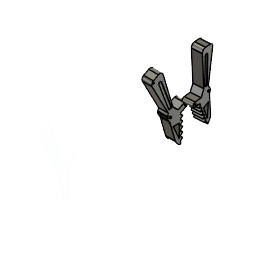
6DOF INDUSTRIAL ROBOTIC ARM (Autodesk Fusion 360 archive; units mm, degrees)
design "JAW 7:1"
part number: 2026-03-04-21-54-08-380
Autodesk Fusion 360 part; units mm, degrees
(part 1 of 2)
sketch "Sketch1" plane through (0, 0, 0) normal (1, 0, 0) x (0, 0, -1)
  line L0 (202.1362, -69.2043) -> (169.6449, -7.2018)
  line L1 (169.6449, -7.2018) -> (190.7116, 4.2958)
  line L2 (190.7116, 4.2958) -> (210.5911, -63.8644)
  line L3 (210.5911, -63.8644) -> (202.1362, -69.2043)
  line L4 (202.1362, -69.2043) -> (200.5414, -75)
  line L5 (200.5414, -75) -> (200.5414, -78.3577)
  line L6 (200.5414, -78.3577) -> (205, -85)
  line L7 (205, -85) -> (215, -120)
  line L8 (215, -120) -> (215, -130)
  line L9 (215, -130) -> (225, -130)
  line L10 (225, -130) -> (225, -80)
  line L11 (225, -80) -> (235, -75)
  line L12 (210.5911, -63.8644) -> (220, -72.7707)
  line L13 (220, -72.7707) -> (231.4715, -67.0349)
  arc A0 (235, -75) -> (231.1083, -67.2166) centre (233.2358, -71.0175) ccw
  dimension "d8" = 70
  dimension "d9" = 24
  dimension "d10" = 71
  dimension "d11" = 15
  dimension "d12" = 10
  dimension "d14" = 10
  dimension "d15" = 8
  dimension "d19" = 8.7116
  constraint vertical L5
  constraint vertical L8
  constraint perpendicular L8 L9
  constraint perpendicular L9 L10
  constraint parallel L11 L13
  constraint coincident L13.end A0
  constraint coincident L13 A0.end
  measures "d8" distance of L0.start L0.end
  measures "d9" distance of L0.end L1.end
  measures "d10" distance of L2.end L1.end
  measures "d11" distance of L2.end L4.end
  measures "d12" distance of L0.start L2.end
  measures "d14" vertical distance of L4.end L6.end
  measures "d15" distance of L5.end L6.end
  measures "d19" distance of L11.end L13.end
extrude "Extrude1" add sketch "Sketch1" along normal mid plane 18 contours L0 L1 L2 L3 | L3 L4 L5 L6 L7 L8 L9 L10 L11 L12 L13 A0 makes body 1
sketch "Sketch2" plane through (-9, 0, 0) normal (-1, 0, 0) x (0, 0, 1)
  line L0 (-200.5414, -75) -> (-202.1362, -69.2043)
  line L1 (-202.1362, -69.2043) -> (-169.6449, -7.2018)
  line L2 (-169.6449, -7.2018) -> (-190.7116, 4.2958)
  line L3 (-190.7116, 4.2958) -> (-210.5911, -63.8644)
  line L4 (-210.5911, -63.8644) -> (-220, -72.7707)
  line L5 (-220, -72.7707) -> (-231.4715, -67.0349)
  arc A0 (-231.4715, -67.0349) -> (-235, -75) centre (-233.2358, -71.0175) ccw
  line L6 (-235, -75) -> (-225, -80)
  line L7 (-225, -80) -> (-225, -130)
  line L8 (-225, -130) -> (-215, -130)
  line L9 (-215, -130) -> (-215, -120)
  line L10 (-215, -120) -> (-205, -85)
  line L11 (-205, -85) -> (-200.5414, -78.3577)
  line L12 (-200.5414, -78.3577) -> (-200.5414, -75)
sketch "Sketch3" plane through (9, 0, 0) normal (1, 0, 0) x (0, 0, -1)
  line L0 (202.1362, -69.2043) -> (200.5414, -75)
  line L1 (200.5414, -75) -> (200.5414, -78.3577)
  line L2 (200.5414, -78.3577) -> (205, -85)
  line L3 (205, -85) -> (215, -120)
  line L4 (215, -120) -> (215, -130)
  line L5 (215, -130) -> (225, -130)
  line L6 (225, -130) -> (225, -80)
  line L7 (225, -80) -> (235, -75)
  arc A0 (235, -75) -> (231.4715, -67.0349) centre (233.2358, -71.0175) ccw
  line L8 (231.4715, -67.0349) -> (220, -72.7707)
  line L9 (220, -72.7707) -> (210.5911, -63.8644)
  line L10 (210.5911, -63.8644) -> (190.7116, 4.2958)
  line L11 (190.7116, 4.2958) -> (169.6449, -7.2018)
  line L12 (169.6449, -7.2018) -> (202.1362, -69.2043)
  line L13 (215, -120) -> (222.3, -120)
  line L14 (222.3, -120) -> (222.3, -95)
  line L15 (222.3, -95) -> (211.3, -95)
  line L16 (211.3, -95) -> (222.3, -120)
  dimension "d23" = 25
  dimension "d24" = 11
  dimension "d25" = 2.7
  constraint coincident L3.end L4.start
  constraint perpendicular L4 L13
  constraint perpendicular L13 L14
  constraint perpendicular L14 L15
  measures "d23" distance of L13.end L14.end
  measures "d24" distance of L14.end L15.end
  measures "d25" distance of L6 L14
extrude "Extrude2" cut sketch "Sketch3" against normal blind 37 contours L14 L15 L16 bodies 1
sketch "Sketch4" plane through (9, 0, 0) normal (1, 0, 0) x (0, 0, -1)
  line L0 (222.3, -95) -> (222.3, -120)
  line L1 (222.3, -120) -> (211.3, -95)
  line L2 (211.3, -95) -> (222.3, -95)
  line L3 (202.1362, -69.2043) -> (200.5414, -75)
  line L4 (200.5414, -75) -> (200.5414, -78.3577)
  line L5 (200.5414, -78.3577) -> (205, -85)
  line L6 (205, -85) -> (215, -120)
  line L7 (215, -120) -> (215, -130)
  line L8 (215, -130) -> (225, -130)
  line L9 (225, -130) -> (225, -80)
  line L10 (225, -80) -> (235, -75)
  arc A0 (235, -75) -> (231.4715, -67.0349) centre (233.2358, -71.0175) ccw
  line L11 (231.4715, -67.0349) -> (220, -72.7707)
  line L12 (220, -72.7707) -> (210.5911, -63.8644)
  line L13 (210.5911, -63.8644) -> (190.7116, 4.2958)
  line L14 (190.7116, 4.2958) -> (169.6449, -7.2018)
  line L15 (169.6449, -7.2018) -> (202.1362, -69.2043)
  line L16 (225, -130) -> (225, -125)
  line L17 (225, -125) -> (225, -121)
  line L18 (225, -121) -> (229, -121)
  line L19 (225, -118) -> (229, -121)
  line L20 (229, -121) -> (225, -124)
  line L21 (225, -109.25) -> (229, -112.25)
  line L22 (229, -112.25) -> (225, -115.25)
  line L23 (225, -100.5) -> (229, -103.5)
  line L24 (229, -103.5) -> (225, -106.5)
  line L25 (225, -91.75) -> (229, -94.75)
  line L26 (229, -94.75) -> (225, -97.75)
  line L27 (225, -83) -> (229, -86)
  line L28 (229, -86) -> (225, -89)
  dimension "d28" = 5
  dimension "d29" = 4
  dimension "d30" = 4
  dimension "d35" = 0
  dimension "d36" = 35
  constraint coincident L8.end L9.start
  constraint perpendicular L8 L16
  constraint parallel L9 L17
  constraint perpendicular L9 L18
  constraint coincident L9 L19.start
  constraint coincident L9 L20.end
  measures "d28" distance of L8.end L16.end
  measures "d29" distance of L16.end L17.end
  measures "d30" distance of L17.end L18.end
extrude "Extrude3" add sketch "Sketch4" against normal up to surface (18 mm away) contours L9 L17 L18 L20 | L9 L18 L19 bodies 1
extrude "Extrude4" add sketch "Sketch4" against normal up to surface (18 mm away) contours L9 L27 L28 | L9 L25 L26 | L9 L21 L22 | L9 L23 L24 bodies 1
fillet "Fillet1" radius 6 2 edges at (0, 4.2958, -190.7116) (0, -7.2018, -169.6449) on bodies 1
fillet "Fillet2" radius 15 1 edges at (0, -130, -215) on bodies 1
fillet "Fillet3" radius 7.5 2 edges at (0, -75, -200.5414) (0, -78.3577, -200.5414) on bodies 1
sketch "Sketch5" plane through (9, 0, 0) normal (1, 0, 0) x (0, 0, -1)
  arc A0 (200.5414, -76.0739) -> (201.8142, -80.2539) centre (208.0414, -76.0739) ccw
  line L0 (201.8142, -80.2539) -> (205, -85)
  line L1 (205, -85) -> (215, -120)
  arc A1 (215, -120) -> (225, -130) centre (229.3541, -115.6459) ccw
  line L2 (225, -130) -> (225, -124)
  line L3 (225, -124) -> (229, -121)
  line L4 (229, -121) -> (225, -118)
  line L5 (225, -118) -> (225, -115.25)
  line L6 (225, -115.25) -> (229, -112.25)
  line L7 (229, -112.25) -> (225, -109.25)
  line L8 (225, -109.25) -> (225, -106.5)
  line L9 (225, -106.5) -> (229, -103.5)
  line L10 (229, -103.5) -> (225, -100.5)
  line L11 (225, -100.5) -> (225, -97.75)
  line L12 (225, -97.75) -> (229, -94.75)
  line L13 (229, -94.75) -> (225, -91.75)
  line L14 (225, -91.75) -> (225, -89)
  line L15 (225, -89) -> (229, -86)
  line L16 (229, -86) -> (225, -83)
  line L17 (225, -83) -> (225, -80)
  line L18 (225, -80) -> (235, -75)
  arc A2 (235, -75) -> (231.4715, -67.0349) centre (233.2358, -71.0175) ccw
  line L19 (231.4715, -67.0349) -> (220, -72.7707)
  line L20 (220, -72.7707) -> (210.5911, -63.8644)
  line L21 (210.5911, -63.8644) -> (192.7997, -2.8637)
  arc A3 (192.7997, -2.8637) -> (184.1653, 0.723) centre (187.0397, -4.5436) ccw
  line L22 (184.1653, 0.723) -> (174.8233, -4.3755)
  arc A4 (174.8233, -4.3755) -> (172.3832, -12.4272) centre (177.6977, -9.6422) ccw
  line L23 (172.3832, -12.4272) -> (202.1362, -69.2043)
  line L24 (202.1362, -69.2043) -> (200.8102, -74.0232)
  arc A5 (200.8102, -74.0232) -> (200.5414, -76.0131) centre (208.0414, -76.0131) ccw
  line L25 (200.5414, -76.0131) -> (200.5414, -76.0739)
  line L26 (222.3, -95) -> (222.3, -120)
  line L27 (222.3, -120) -> (211.3, -95)
  line L28 (211.3, -95) -> (222.3, -95)
  circle A6 centre (175, -8) radius 1.4142
extrude "Extrude5" cut sketch "Sketch5" against normal blind 15 contours A6 bodies 1
sketch "Sketch6" plane through (0, 47.7358, -167.0755) normal (0, -0.274721, 0.961524) x (1, 0, 0)
  line L0 (-9, -174.4479) -> (9, -174.4479)
  line L1 (9, -174.4479) -> (9, -138.0474)
  line L2 (9, -138.0474) -> (-9, -138.0474)
  line L3 (-9, -138.0474) -> (-9, -174.4479)
  line L4 (-6.0554, -142) -> (6.0554, -142)
  line L5 (-9, -138.0474) -> (-9, -141.4259)
  line L6 (9, -138.0474) -> (9, -141.4259)
  line L7 (-6.0232, -143.0955) -> (6.0232, -143.0955)
  line L8 (-6.0554, -142) -> (-6.0232, -143.0955)
  line L9 (6.0554, -142) -> (6.0232, -143.0955)
  dimension "d47" = 3
  dimension "d48" = 3
  dimension "d49" = 3.9526
  constraint horizontal L4
  constraint coincident L2.end L3.start
  constraint coincident L3 L5.end
  constraint coincident L1.end L2.start
  constraint coincident L1 L6.end
  constraint parallel L0 L7
  measures "d47" distance of L4.end L6.end
  measures "d48" distance of L4.start L5.end
  measures "d49" distance of L2 L4
extrude "Extrude6" cut sketch "Sketch6" against normal blind 10 contours L4 L7 L8 L9 bodies 1
sketch "Sketch7" plane through (9, 0, 0) normal (1, 0, 0) x (0, 0, -1)
  circle A0 centre (175, -8) radius 1.4142
  arc A1 (200.5414, -76.0739) -> (201.8142, -80.2539) centre (208.0414, -76.0739) ccw
  line L0 (201.8142, -80.2539) -> (205, -85)
  line L1 (205, -85) -> (215, -120)
  arc A2 (215, -120) -> (225, -130) centre (229.3541, -115.6459) ccw
  line L2 (225, -130) -> (225, -124)
  line L3 (225, -124) -> (229, -121)
  line L4 (229, -121) -> (225, -118)
  line L5 (225, -118) -> (225, -115.25)
  line L6 (225, -115.25) -> (229, -112.25)
  line L7 (229, -112.25) -> (225, -109.25)
  line L8 (225, -109.25) -> (225, -106.5)
  line L9 (225, -106.5) -> (229, -103.5)
  line L10 (229, -103.5) -> (225, -100.5)
  line L11 (225, -100.5) -> (225, -97.75)
  line L12 (225, -97.75) -> (229, -94.75)
  line L13 (229, -94.75) -> (225, -91.75)
  line L14 (225, -91.75) -> (225, -89)
  line L15 (225, -89) -> (229, -86)
  line L16 (229, -86) -> (225, -83)
  line L17 (225, -83) -> (225, -80)
  line L18 (225, -80) -> (235, -75)
  arc A3 (235, -75) -> (231.4715, -67.0349) centre (233.2358, -71.0175) ccw
  line L19 (231.4715, -67.0349) -> (220, -72.7707)
  line L20 (220, -72.7707) -> (210.5911, -63.8644)
  line L21 (210.5911, -63.8644) -> (192.7997, -2.8637)
  arc A4 (192.7997, -2.8637) -> (184.1653, 0.723) centre (187.0397, -4.5436) ccw
  line L22 (184.1653, 0.723) -> (174.8233, -4.3755)
  arc A5 (174.8233, -4.3755) -> (172.3832, -12.4272) centre (177.6977, -9.6422) ccw
  line L23 (172.3832, -12.4272) -> (202.1362, -69.2043)
  line L24 (202.1362, -69.2043) -> (200.8102, -74.0232)
  arc A6 (200.8102, -74.0232) -> (200.5414, -76.0131) centre (208.0414, -76.0131) ccw
  line L25 (200.5414, -76.0131) -> (200.5414, -76.0739)
  line L26 (222.3, -95) -> (222.3, -120)
  line L27 (222.3, -120) -> (211.3, -95)
  line L28 (211.3, -95) -> (222.3, -95)
  circle A7 centre (233.2358, -71.0175) radius 1.75
  circle A8 centre (205, -77) radius 1.75
  dimension "d52" = 3.5
  dimension "d53" = 3.5
  constraint concentric A3 A7
  measures "d52" diameter of A7
  measures "d53" diameter of A8
extrude "Extrude7" add sketch "Sketch7" along normal blind 1.5 contours A7 | A8 bodies 1
sketch "Sketch8" plane through (9, 0, 0) normal (1, 0, 0) x (0, 0, -1)
  circle A0 centre (205, -77) radius 1.75
  circle A1 centre (233.2358, -71.0175) radius 1.75
  circle A2 centre (175, -8) radius 1.4142
  arc A3 (200.5414, -76.0739) -> (201.8142, -80.2539) centre (208.0414, -76.0739) ccw
  line L0 (201.8142, -80.2539) -> (205, -85)
  line L1 (205, -85) -> (215, -120)
  arc A4 (215, -120) -> (225, -130) centre (229.3541, -115.6459) ccw
  line L2 (225, -130) -> (225, -124)
  line L3 (225, -124) -> (229, -121)
  line L4 (229, -121) -> (225, -118)
  line L5 (225, -118) -> (225, -115.25)
  line L6 (225, -115.25) -> (229, -112.25)
  line L7 (229, -112.25) -> (225, -109.25)
  line L8 (225, -109.25) -> (225, -106.5)
  line L9 (225, -106.5) -> (229, -103.5)
  line L10 (229, -103.5) -> (225, -100.5)
  line L11 (225, -100.5) -> (225, -97.75)
  line L12 (225, -97.75) -> (229, -94.75)
  line L13 (229, -94.75) -> (225, -91.75)
  line L14 (225, -91.75) -> (225, -89)
  line L15 (225, -89) -> (229, -86)
  line L16 (229, -86) -> (225, -83)
  line L17 (225, -83) -> (225, -80)
  line L18 (225, -80) -> (235, -75)
  arc A5 (235, -75) -> (231.4715, -67.0349) centre (233.2358, -71.0175) ccw
  line L19 (231.4715, -67.0349) -> (220, -72.7707)
  line L20 (220, -72.7707) -> (210.5911, -63.8644)
  line L21 (210.5911, -63.8644) -> (192.7997, -2.8637)
  arc A6 (192.7997, -2.8637) -> (184.1653, 0.723) centre (187.0397, -4.5436) ccw
  line L22 (184.1653, 0.723) -> (174.8233, -4.3755)
  arc A7 (174.8233, -4.3755) -> (172.3832, -12.4272) centre (177.6977, -9.6422) ccw
  line L23 (172.3832, -12.4272) -> (202.1362, -69.2043)
  line L24 (202.1362, -69.2043) -> (200.8102, -74.0232)
  arc A8 (200.8102, -74.0232) -> (200.5414, -76.0131) centre (208.0414, -76.0131) ccw
  line L25 (200.5414, -76.0131) -> (200.5414, -76.0739)
  line L26 (222.3, -95) -> (222.3, -120)
  line L27 (222.3, -120) -> (211.3, -95)
  line L28 (211.3, -95) -> (222.3, -95)
  line L29 (184.9185, -15.1863) -> (202.539, -62.9087)
  arc A9 (202.539, -62.9087) -> (207.461, -61.0913) centre (205, -62) ccw
  line L30 (207.461, -61.0913) -> (189.8405, -13.3689)
  arc A10 (189.8405, -13.3689) -> (184.9185, -15.1863) centre (187.3795, -14.2776) ccw
  line L31 (187.3795, -14.2776) -> (205, -62) construction
  constraint tangent L29 A9
  constraint tangent A9 L30
  constraint parallel L29 L30
  constraint tangent L30 A10
  constraint tangent L29 A10
extrude "Extrude8" cut sketch "Sketch8" against normal blind 1 contours L29 A9 L30 A10 bodies 1
ref_plane "WorkPlane1" through (0, -62.8521, -204.3137) normal (1, 0, 0) x (0, 0, -1)
mirror "Mirror1" about plane through (0, -62.8521, -204.3137) normal (1, 0, 0) of "Extrude7", "Extrude8"
move_body "Move1" bodies 1 to x (1, 0, 0) y (0, 1, 0) z (0, 0, 1) at (-1.5949, 0, 1.5335)
extrude "Extrude9" add 1 faces at (-3.6026, -88.9381, -208.0584) along direction (0, 0.961524, 0.274721) blind 2 on bodies 1 bodies 1
copy_body "CopyPasteBodies3" bodies 1 makes body 2
move_body "Move4" bodies 2 to x (-0.987971, 0.068961, 0.138413) y (0.119618, 0.908062, 0.401392) z (-0.098007, 0.41312, -0.905387) at (56.4118, 154.4, -545.695)
move_body "Move5" bodies 1 to x (1, 0, 0) y (0, 1, 0) z (0, 0, 1) at (60, 60, -130)

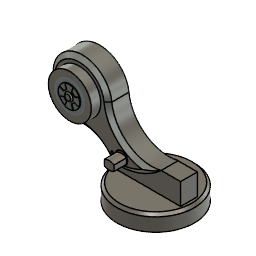
design "PART 2"
part number: 2026-02-23-03-24-46-902
Autodesk Fusion 360 part; units mm, degrees
sketch "Sketch1" plane through (0, 0, 0) normal (0, 1, 0) x (1, 0, 0)
  circle A0 centre (0, 0) radius 90
  dimension "d1" = 180
  constraint coincident A0.centre origin
  measures "d1" diameter of A0
extrude "Extrude1" add sketch "Sketch1" along normal blind 37 makes body 1
chamfer "Chamfer1" distance 6 angle 45 1 edges at (-83.9095, 37, 32.5454) on bodies 1
sketch "Sketch2" plane through (0, 37, 0) normal (0, 1, 0) x (-1, 0, 0)
  circle A0 centre (0, 0) radius 84
  line L0 (-77.5, 19.5) -> (77.5, 19.5)
  line L1 (77.5, 19.5) -> (77.5, -19.5)
  line L2 (77.5, -19.5) -> (-77.5, -19.5)
  line L3 (-77.5, -19.5) -> (-77.5, 19.5)
  line L4 (-77.5, 19.5) -> (77.5, -19.5) construction
  line L5 (77.5, 19.5) -> (-77.5, -19.5) construction
  dimension "d5" = 39
  dimension "d6" = 155
  constraint horizontal L0
  constraint perpendicular L0 L1
  constraint parallel L0 L2
  constraint parallel L1 L3
  constraint coincident L4 A0.centre
  constraint coincident L5 A0.centre
  constraint coincident A0.centre origin
  measures "d5" distance of L0.end L1.end
  measures "d6" distance of L1.end L2.end
extrude "Extrude2" add sketch "Sketch2" along normal blind 50 contours L0 L1 L2 L3 bodies 1
sketch "Sketch3" plane through (0, 0, 19.5) normal (0, 0, 1) x (1, 0, 0)
  line L0 (-77.5, 37) -> (77.5, 37)
  line L1 (77.5, 37) -> (77.5, 87)
  line L2 (77.5, 87) -> (-77.5, 87)
  line L3 (-77.5, 87) -> (-77.5, 37)
  line L4 (-77.5, 87) -> (32.5, 87)
  line L5 (-77.5, 87) -> (-77.5, 48)
  arc A0 (-77.5, 48) -> (32.5, 87) centre (-68.6761, 197.7402) ccw
  dimension "d9" = 110
  dimension "d10" = 39
  dimension "d11" = 150
  constraint coincident L2.end L3.start
  constraint coincident L2 L4.end
  constraint perpendicular L2 L5
  measures "d9" distance of L2.end L4.end
  measures "d10" distance of L2.end L5.end
  measures "d11" radius of A0
extrude "Extrude3" cut sketch "Sketch3" against normal blind 100 contours L2 L3 L4 L5 A0 bodies 1
sketch "Sketch4" plane through (0, 0, 0) normal (0, 0, 1) x (1, 0, 0)
  line L0 (0, 0) -> (-150, 0)
  line L1 (-150, 0) -> (-150, 160)
  circle A0 centre (-150, 160) radius 68.5
  arc A1 (-81.9123, 167.5039) -> (32.5, 87) centre (10.8064, 177.7224) ccw
  arc A2 (-77.5, 48) -> (-150, 91.5) centre (-150, 9.3333) ccw
  arc A3 (-77.5, 48) -> (32.5, 87) centre (-69.9351, 201.2914) ccw
  dimension "d14" = 150
  dimension "d15" = 160
  dimension "d16" = 137
  constraint coincident L0.start origin
  constraint horizontal L0
  constraint perpendicular L0 L1
  constraint coincident L1.end A0.centre
  constraint tangent A0 A1
  constraint coincident A0 A1.start
  constraint tangent A0 A2
  constraint coincident A0 A2.end
  constraint coincident L1 A2.end
  measures "d14" distance of L0.start L0.end
  measures "d15" distance of L0.end L1.end
  measures "d16" diameter of A0
extrude "Extrude4" add sketch "Sketch4" along normal mid plane 40 bodies 1
sketch "Sketch5" plane through (0, 0, 0) normal (0, 0, 1) x (1, 0, 0)
  arc A0 (-77.5, 48) -> (-150, 91.5) centre (-150, 9.3333) ccw
  arc A1 (-81.9123, 167.5039) -> (32.5, 87) centre (10.8064, 177.7224) ccw
  circle A2 centre (-150, 160) radius 68.5
  arc A3 (-77.5, 48) -> (32.5, 87) centre (-68.6761, 197.7402) ccw
extrude "Extrude5" add 1 faces at (-157.7558, 155.7766, 20) along direction (0, 0, 1) blind 7.5 draft -55 on bodies 1 bodies 1
sketch "Sketch6" plane through (0, 0, 27.5) normal (0, 0, 1) x (1, 0, 0)
  arc A0 (-92.5589, 166.3306) -> (-150, 102.2111) centre (-150, 160) ccw
  arc A1 (-71.2223, 58.5304) -> (-150, 102.2111) centre (-150, 9.3333) ccw
  arc A2 (-71.2223, 58.5304) -> (-3.8068, 74.7631) centre (-69.9351, 201.2914) ccw
  arc A3 (-92.5589, 166.3306) -> (-3.8068, 74.7631) centre (10.8064, 177.7224) ccw
  circle A4 centre (-150, 160) radius 50
  dimension "d21" = 100
  constraint concentric A0 A4
  measures "d21" diameter of A4
extrude "Extrude6" add sketch "Sketch6" along normal blind 3 contours A4 bodies 1
extrude "Extrude7" add 1 faces at (-167.3965, 167.9656, 30.5) along direction (0, 0, 1) blind 19 draft -40 on bodies 1 bodies 1
sketch "Sketch7" plane through (0, 0, 49.5) normal (0, 0, 1) x (1, 0, 0)
  circle A0 centre (-150, 160) radius 34.0571
sketch "Sketch8" plane through (0, 0, -20) normal (0, 0, -1) x (-1, 0, 0)
  arc A0 (150, 91.5) -> (81.9123, 167.5039) centre (150, 160) ccw
  arc A1 (-32.5, 87) -> (81.9123, 167.5039) centre (-10.8064, 177.7224) ccw
  arc A2 (-32.5, 87) -> (77.5, 48) centre (69.9351, 201.2914) ccw
  arc A3 (150, 91.5) -> (77.5, 48) centre (150, 9.3333) ccw
sketch "Sketch9" plane through (0, 0, 49.5) normal (0, 0, 1) x (1, 0, 0)
delete_face "DeleteFace1" 1 faces at (-133.6745, 118.4033, 36.8333) on bodies 1
sketch "Sketch10" plane through (0, 0, 0) normal (0, 0, 1) x (1, 0, 0)
sketch "Sketch11" plane through (0, 0, 0) normal (0, 0, 1) x (1, 0, 0)
sketch "Sketch12" plane through (0, 0, 0) normal (0, 0, 1) x (1, 0, 0)
sketch "Sketch13" plane through (0, 0, 49.5) normal (0, 0, 1) x (1, 0, 0)
sketch "Sketch14" plane through (0, 0, 49.5) normal (0, 0, 1) x (1, 0, 0)
  circle A0 centre (-150, 160) radius 13
  circle A1 centre (-150, 160) radius 25
  dimension "d31" = 26
  dimension "d32" = 50
  constraint concentric A0 A1
  measures "d31" diameter of A0
  measures "d32" diameter of A1
extrude "Extrude8" add sketch "Sketch14" along normal blind 1 separate body contours A0 | A1 makes body 2
sketch "Sketch15" plane through (0, 0, 50.5) normal (0, 0, 1) x (1, 0, 0)
  circle A0 centre (-150, 160) radius 25
  circle A1 centre (-150, 160) radius 13
  line L0 (-159.5509, 183.1037) -> (-155.4394, 171.8073)
  line L1 (-140.4491, 183.1037) -> (-144.5606, 171.8073)
  line L2 (-173.1037, 150.4491) -> (-161.8073, 154.5606)
  line L3 (-173.1037, 169.5509) -> (-161.8073, 165.4394)
  line L4 (-140.4491, 136.8963) -> (-144.5606, 148.1927)
  line L5 (-159.5509, 136.8963) -> (-155.4394, 148.1927)
  line L6 (-126.8963, 169.5509) -> (-138.1927, 165.4394)
  line L7 (-126.8963, 150.4491) -> (-138.1927, 154.5606)
  dimension "d35" = 26
  dimension "d38" = 360
  constraint concentric A0 A1
  constraint coincident A0 L0.start
  constraint coincident A1 L0.end
  measures "d35" diameter of A1
extrude "Extrude9" add sketch "Sketch15" along normal blind 1 contours A0 A1 L6 L7 | A0 A1 L0 L1 | A1 | A0 A1 L4 L5 | A0 A1 L2 L3 bodies 2
sketch "Sketch16" plane through (0, 0, 51.5) normal (0, 0, 1) x (1, 0, 0)
  line L0 (-126.8963, 169.5509) -> (-138.1927, 165.4394)
  arc A0 (-138.1927, 165.4394) -> (-144.5606, 171.8073) centre (-150, 160) ccw
  line L1 (-144.5606, 171.8073) -> (-140.4491, 183.1037)
  arc A1 (-140.4491, 183.1037) -> (-159.5509, 183.1037) centre (-150, 160) ccw
  line L2 (-159.5509, 183.1037) -> (-155.4394, 171.8073)
  arc A2 (-155.4394, 171.8073) -> (-161.8073, 165.4394) centre (-150, 160) ccw
  line L3 (-161.8073, 165.4394) -> (-173.1037, 169.5509)
  arc A3 (-173.1037, 169.5509) -> (-173.1037, 150.4491) centre (-150, 160) ccw
  line L4 (-173.1037, 150.4491) -> (-161.8073, 154.5606)
  arc A4 (-161.8073, 154.5606) -> (-155.4394, 148.1927) centre (-150, 160) ccw
  line L5 (-155.4394, 148.1927) -> (-159.5509, 136.8963)
  arc A5 (-159.5509, 136.8963) -> (-140.4491, 136.8963) centre (-150, 160) ccw
  line L6 (-140.4491, 136.8963) -> (-144.5606, 148.1927)
  arc A6 (-144.5606, 148.1927) -> (-138.1927, 154.5606) centre (-150, 160) ccw
  line L7 (-138.1927, 154.5606) -> (-126.8963, 150.4491)
  arc A7 (-126.8963, 150.4491) -> (-126.8963, 169.5509) centre (-150, 160) ccw
  circle A8 centre (-150, 160) radius 9.5
  dimension "d41" = 19
  constraint concentric A0 A8
  measures "d41" diameter of A8
extrude "Extrude10" add sketch "Sketch16" along normal blind 3 draft -45 contours A8 bodies 2
sketch "Sketch17" plane through (0, 0, 27.5) normal (0, 0, 1) x (1, 0, 0)
  circle A0 centre (-150, 160) radius 50
  arc A1 (-92.5589, 166.3306) -> (-150, 102.2111) centre (-150, 160) ccw
  arc A2 (-71.2223, 58.5304) -> (-150, 102.2111) centre (-150, 9.3333) ccw
  arc A3 (-71.2223, 58.5304) -> (-3.8068, 74.7631) centre (-69.9351, 201.2914) ccw
  arc A4 (-92.5589, 166.3306) -> (-3.8068, 74.7631) centre (10.8064, 177.7224) ccw
  line L0 (-63.2112, 80.0232) -> (-40.2112, 80.0232)
  line L1 (-40.2112, 80.0232) -> (-40.2112, 67.0232)
  line L2 (-40.2112, 67.0232) -> (-63.2112, 67.0232)
  line L3 (-63.2112, 67.0232) -> (-63.2112, 80.0232)
  arc A5 (-40.2112, 80.0232) -> (-63.2112, 80.0232) centre (-51.7112, 60.1046) ccw
  arc A6 (-63.2112, 67.0232) -> (-40.2112, 67.0232) centre (-51.7112, 86.9417) ccw
  dimension "d44" = 23
  dimension "d45" = 13
  dimension "d46" = 23
  dimension "d47" = 23
  constraint horizontal L0
  constraint vertical L1
  constraint horizontal L2
  constraint vertical L3
  measures "d44" distance of L0.start L0.end
  measures "d45" distance of L0.start L2.end
  measures "d46" radius of A5
  measures "d47" radius of A6
extrude "Extrude11" add sketch "Sketch17" along normal blind 22 separate body contours L0 A5 | L0 L1 L2 L3 | L2 A6 makes body 3
sketch "Sketch18" plane through (0, 0, 49.5) normal (0, 0, 1) x (1, 0, 0)
  arc A0 (-40.2112, 80.0232) -> (-63.2112, 80.0232) centre (-51.7112, 60.1046) ccw
  line L0 (-63.2112, 80.0232) -> (-63.2112, 67.0232)
  arc A1 (-63.2112, 67.0232) -> (-40.2112, 67.0232) centre (-51.7112, 86.9417) ccw
  line L1 (-40.2112, 67.0232) -> (-40.2112, 80.0232)
  line L2 (-40.2112, 67.0232) -> (-40.2112, 80.0232)
  arc A2 (-40.2112, 80.0232) -> (-63.2112, 80.0232) centre (-51.7112, 60.1046) ccw
  line L3 (-63.2112, 80.0232) -> (-63.2112, 67.0232)
  arc A3 (-63.2112, 67.0232) -> (-40.2112, 67.0232) centre (-51.7112, 86.9417) ccw
  line L4 (-41.8196, 67.9745) -> (-41.8196, 79.0718)
  arc A4 (-41.8196, 79.0718) -> (-61.6028, 79.0718) centre (-51.7112, 60.1046) ccw
  line L5 (-61.6028, 79.0718) -> (-61.6028, 67.9745)
  arc A5 (-61.6028, 67.9745) -> (-41.8196, 67.9745) centre (-51.7112, 86.9417) ccw
  dimension "d52" = 0
  dimension "d53" = -1.6084
  measures "d52" distance of L0
extrude "Extrude12" add sketch "Sketch18" along normal blind 7 contours A0 L0 A1 L1 L2 A2 L3 A3 | L4 A4 L5 A5 bodies 3
sketch "Sketch19" plane through (0, 0, 27.5) normal (0, 0, 1) x (1, 0, 0)
  circle A0 centre (-150, 160) radius 50
  arc A1 (-92.5589, 166.3306) -> (-150, 102.2111) centre (-150, 160) ccw
  arc A2 (-71.2223, 58.5304) -> (-150, 102.2111) centre (-150, 9.3333) ccw
  arc A3 (-71.2223, 58.5304) -> (-3.8068, 74.7631) centre (-69.9351, 201.2914) ccw
  arc A4 (-92.5589, 166.3306) -> (-3.8068, 74.7631) centre (10.8064, 177.7224) ccw
  line L0 (-40, 80) -> (-63, 67)
  circle A5 centre (-52, 74) radius 13.8924
  circle A6 centre (-52, 74) radius 14.4222
  circle A7 centre (-73.4038, 74) radius 2.4435
  circle A8 centre (-73.4038, 74) radius 3.127
  constraint concentric A5 A6
  constraint concentric A7 A8
extrude "Extrude13" cut sketch "Sketch19" against normal blind 0.9 contours A3 A6 | A8 picked at (-66.0042, 75.0445) bodies 1
sketch "Sketch20" plane through (0, 0, 0) normal (0, -1, 0) x (1, 0, 0)
  circle A0 centre (0, 0) radius 90
  circle A1 centre (0, 0) radius 15
  dimension "d56" = 30
  constraint concentric A0 A1
  measures "d56" diameter of A1
extrude "Extrude14" cut sketch "Sketch20" against normal blind 20 contours A1 bodies 1
sketch "Sketch21" plane through (0, 0, -20) normal (0, 0, -1) x (-1, 0, 0)
  circle A0 centre (150, 175) radius 15
  dimension "d59" = 30
  measures "d59" diameter of A0
extrude "Extrude15" cut sketch "Sketch21" against normal blind 20 bodies 1
named bodies: "JAW1"

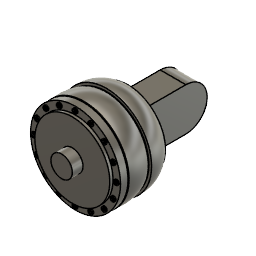
design "JAW 5:1"
part number: 2026-03-04-08-28-14-170
Autodesk Fusion 360 part; units mm, degrees
sketch "Sketch1" plane through (0, 0, 0) normal (0, 1, 0) x (1, 0, 0)
  line L0 (0, 0) -> (-35, 0)
  line L1 (0, 0) -> (0, -20)
  line L2 (0, -20) -> (-42, -20)
  arc A0 (-35, 0) -> (-42, -20) centre (-17.1273, -17.4804) ccw
  dimension "d2" = 20
  dimension "d3" = 42
  dimension "d4" = 25
  constraint coincident L0.start L1.start
  constraint horizontal L0
  constraint perpendicular L0 L1
  constraint perpendicular L1 L2
  measures "d2" distance of L0.start L1.end
  measures "d3" distance of L1.end L2.end
  measures "d4" radius of A0
revolve "Revolve1" add sketch "Sketch1" angle 360 about axis through (0, 0, 0) along (0, 0, 1) makes body 1
sketch "Sketch2" plane through (0, 0, 20) normal (0, 0, 1) x (1, 0, 0)
  circle A0 centre (0, 0) radius 42
  circle A1 centre (0, 0) radius 39.5
  dimension "d6" = 79
  constraint coincident A0.centre A1.centre
  measures "d6" diameter of A1
extrude "Extrude1" add sketch "Sketch2" along normal blind 1 contours A1 bodies 1
sketch "Sketch3" plane through (0, 0, 0) normal (0, 1, 0) x (1, 0, 0)
sketch "Sketch4" plane through (0, 0, 0) normal (0, 1, 0) x (1, 0, 0)
  line L0 (0, -21) -> (0, -41)
  line L1 (0, -21) -> (-39.5, -21)
  line L2 (0, -21) -> (-40, -21)
  line L3 (0, -41) -> (-42, -41)
  arc A0 (-40, -21) -> (-42, -41) centre (-5.5677, -34.5432) ccw
  dimension "d13" = 20
  dimension "d14" = 40
  dimension "d15" = 42
  dimension "d17" = 37
  constraint vertical L0
  constraint perpendicular L0 L1
  constraint perpendicular L0 L2
  constraint perpendicular L0 L3
  measures "d13" distance of L0.start L0.end
  measures "d14" distance of L0.start L2.end
  measures "d15" distance of L0.end L3.end
  measures "d17" radius of A0
revolve "Revolve2" add sketch "Sketch4" angle 360 about axis through (0, 0, 21) along (0, 0, 1) bodies 1
sketch "Sketch5" plane through (0, 0, 41) normal (0, 0, 1) x (1, 0, 0)
  circle A0 centre (0, 0) radius 42
  circle A1 centre (0, 0) radius 41.25
  dimension "d19" = 82.5
  constraint coincident A0.centre A1.centre
  measures "d19" diameter of A1
extrude "Extrude2" add sketch "Sketch5" along normal blind 1 contours A1 bodies 1
sketch "Sketch6" plane through (0, 0, 42) normal (0, 0, 1) x (1, 0, 0)
  circle A0 centre (0, 0) radius 41.25
  circle A1 centre (0, 0) radius 42
  dimension "d22" = 84
  constraint coincident A0.centre A1.centre
  measures "d22" diameter of A1
extrude "Extrude3" add sketch "Sketch6" along normal blind 7 separate body contours A0 | A1 makes body 2
sketch "Sketch7" plane through (0, 0, 49) normal (0, 0, 1) x (1, 0, 0)
  circle A0 centre (0, 0) radius 42
  circle A1 centre (0, 0) radius 35
  dimension "d25" = 70
  constraint concentric A0 A1
  measures "d25" diameter of A1
extrude "Extrude4" add sketch "Sketch7" along normal blind 3 contours A1 bodies 2
sketch "Sketch8" plane through (0, 0, 49) normal (0, 0, 1) x (1, 0, 0)
  circle A0 centre (0, 0) radius 35
  circle A1 centre (0, 0) radius 42
  line L0 (35, 0) -> (42, 0)
  circle A2 centre (38.5, 0) radius 2.25
  circle A3 centre (38.5, 0) radius 1.5
  dimension "d28" = 4.5
  dimension "d29" = 3
  constraint coincident A0 L0.start
  constraint coincident A1 L0.end
  constraint horizontal L0
  constraint midpoint L0 A2.centre
  constraint concentric A2 A3
  measures "d28" diameter of A2
  measures "d29" diameter of A3
extrude "Extrude5" add sketch "Sketch8" along normal blind 1 contours L0 A2 A3 | L0 A2 A3 bodies 2
pattern_circular "C-Pattern1" count 16 over 360 about axis through (0, 0, 52) along (0, 0, 1) of "Extrude5"
sketch "Sketch9" plane through (0, 0, 0) normal (0, 0, -1) x (-1, 0, 0)
  circle A0 centre (0, 0) radius 35
  line L0 (12, -20) -> (-12, -20)
  line L1 (-12, -20) -> (-12, 20)
  line L2 (-12, 20) -> (12, 20)
  line L3 (12, 20) -> (12, -20)
  line L4 (12, -20) -> (-12, 20) construction
  line L5 (-12, -20) -> (12, 20) construction
  dimension "d34" = 40
  dimension "d35" = 24
  constraint horizontal L0
  constraint perpendicular L0 L1
  constraint parallel L0 L2
  constraint parallel L1 L3
  constraint coincident L4 A0.centre
  constraint coincident L5 A0.centre
  constraint coincident A0.centre origin
  measures "d34" distance of L0.start L2.end
  measures "d35" distance of L1.end L2.end
extrude "Extrude6" add sketch "Sketch9" along normal blind 42 contours L0 L1 L2 L3 bodies 1
sketch "Sketch10" plane through (-12, 0, 0) normal (-1, 0, 0) x (0, 0, 1)
  line L0 (0, -20) -> (0, 20)
  line L1 (0, 20) -> (-42, 20)
  line L2 (-42, 20) -> (-42, -20)
  line L3 (-42, -20) -> (0, -20)
  circle A0 centre (-42, 0) radius 20
  dimension "d38" = 40
  constraint midpoint L2 A0.centre
  measures "d38" diameter of A0
extrude "Extrude7" add sketch "Sketch10" against normal blind 24 contours L2 A0 picked at (-48.2058, 2.4356) bodies 1
sketch "Sketch11" plane through (-12, 0, 0) normal (-1, 0, 0) x (0, 0, 1)
  line L0 (0, -20) -> (0, 20)
  line L1 (0, 20) -> (-42, 20)
  arc A0 (-42, 20) -> (-42, -20) centre (-42, 0) ccw
  line L2 (-42, -20) -> (0, -20)
  circle A1 centre (-40, 0) radius 10
  dimension "d41" = 20
  measures "d41" diameter of A1
extrude "Extrude8" add sketch "Sketch11" along normal blind 10 contours A1 bodies 1
sketch "Sketch12" plane through (0, 0, 52) normal (0, 0, 1) x (1, 0, 0)
  circle A0 centre (0, 0) radius 35
  circle A1 centre (0, 0) radius 10
  dimension "d44" = 20
  constraint coincident A0.centre A1.centre
  measures "d44" diameter of A1
extrude "Extrude9" add sketch "Sketch12" along normal blind 10 contours A1 bodies 2

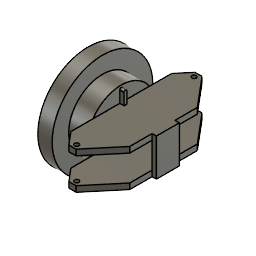
design "JAW 6:1"
part number: 2026-03-04-21-19-51-096
Autodesk Fusion 360 part; units mm, degrees
sketch "Sketch1" plane through (0, 0, 0) normal (1, 0, 0) x (0, 0, -1)
  circle A0 centre (0, 0) radius 35
  dimension "d1" = 70
  constraint coincident A0.centre origin
  measures "d1" diameter of A0
extrude "Extrude1" add sketch "Sketch1" along normal blind 10
sketch "Sketch2" plane through (10, 0, 0) normal (1, 0, 0) x (0, 0, -1)
  circle A0 centre (0, 0) radius 35
  circle A1 centre (0, 0) radius 23.5
  dimension "d4" = 47
  constraint coincident A0.centre A1.centre
  measures "d4" diameter of A1
extrude "Extrude2" add sketch "Sketch2" along normal blind 13 contours A1
ref_plane "WorkPlane1" through (0, 13, 0) normal (0, 1, 0) x (0, 0, 1)
sketch "Sketch3" plane through (0, 13, 0) normal (0, 1, 0) x (1, 0, 0)
  line L0 (23, 0) -> (23, -35)
  line L1 (23, -35) -> (23, -45)
  line L2 (23, -35) -> (30.3921, -43.8095)
  line L3 (30.3921, -43.8095) -> (35.3921, -43.8095)
  line L4 (23, 0) -> (60, 0)
  line L5 (23, -23.5) -> (67, -23.5)
  line L6 (35.3921, -43.8095) -> (52.4338, -23.5)
  line L7 (35.3921, -43.8095) -> (47.3921, -43.8095)
  line L8 (52.4338, -23.5) -> (52.4338, 0)
  line L9 (35.3921, 43.8095) -> (52.4338, 23.5)
  line L10 (30.3921, 43.8095) -> (35.3921, 43.8095)
  line L11 (23, 35) -> (30.3921, 43.8095)
  line L12 (23, 0) -> (23, 35)
  line L13 (52.4338, 0) -> (52.4338, 23.5)
  dimension "d8" = 35
  dimension "d9" = 10
  dimension "d10" = 11.5
  dimension "d11" = 40
  dimension "d12" = 5
  dimension "d13" = 37
  dimension "d14" = 44
  dimension "d15" = 12
  dimension "d16" = 50
  constraint vertical L0
  constraint parallel L0 L1
  constraint horizontal L3
  constraint perpendicular L0 L4
  constraint coincident L0 L5.start
  constraint perpendicular L0 L5
  constraint coincident L5 L6.end
  constraint parallel L3 L7
  constraint coincident L4 L8.end
  constraint perpendicular L4 L8
  constraint symmetric L0.start L4 L12.start
  constraint symmetric L0.end L4 L11.start
  constraint symmetric L2.end L4 L10.start
  constraint symmetric L3.end L4 L9.start
  constraint symmetric L4 L6.end L9.end
  constraint perpendicular L4 L13
  measures "d8" distance of L0.start L0.end
  measures "d9" distance of L0.end L1.end
  measures "d10" distance of L0.end L2.end
  measures "d11" angle of L1 L2
  measures "d12" distance of L2.end L3.end
  measures "d13" distance of L0.start L4.end
  measures "d14" distance of L5.start L5.end
  measures "d15" distance of L3.end L7.end
  measures "d16" angle of L6 L7
extrude "Extrude3" add sketch "Sketch3" against normal blind 4
sketch "Sketch4" plane through (0, 13, 0) normal (0, 1, 0) x (-1, 0, 0)
  line L0 (-23, -35) -> (-23, -19.5768)
  line L1 (-23, -19.5768) -> (-23, 19.5768)
  line L2 (-23, 19.5768) -> (-23, 35)
  line L3 (-23, 35) -> (-30.3921, 43.8095)
  line L4 (-30.3921, 43.8095) -> (-35.3921, 43.8095)
  line L5 (-35.3921, 43.8095) -> (-52.4338, 23.5)
  line L6 (-52.4338, 23.5) -> (-52.4338, -23.5)
  line L7 (-52.4338, -23.5) -> (-35.3921, -43.8095)
  line L8 (-35.3921, -43.8095) -> (-30.3921, -43.8095)
  line L9 (-30.3921, -43.8095) -> (-23, -35)
  line L10 (-32.8921, -43.8095) -> (-32.8921, -40.8095)
  circle A0 centre (-32.8921, -40.8095) radius 1.5
  dimension "d19" = 3
  dimension "d20" = 3
  constraint midpoint L8 L10.start
  constraint perpendicular L8 L10
  constraint coincident L10.end A0.centre
  measures "d19" distance of L10.start L10.end
  measures "d20" diameter of A0
extrude "Extrude4" cut sketch "Sketch4" against normal blind 5 contours A0
mirror "Mirror1" about plane through (0, 0, 0) normal (0, 0, 1) of "Extrude4"
mirror "Mirror2" about plane through (0, 0, 0) normal (0, 1, 0) of "Extrude3", "Extrude4", "Mirror1"
sketch "Sketch5" plane through (23, 0, 0) normal (1, 0, 0) x (0, 0, -1)
  line L0 (-19.5768, 13) -> (19.5768, 13)
  arc A0 (19.5768, 13) -> (-19.5768, 13) centre (0, 0) ccw
  line L1 (0, 13) -> (0, 23.5)
  line L2 (0, 13) -> (-1, 13)
  line L3 (-1, 13) -> (-1, 22)
  line L4 (-1, 22) -> (1, 22)
  line L5 (1, 22) -> (1, 13)
  line L6 (1, 13) -> (0, 13)
  dimension "d27" = 1
  dimension "d28" = 9
  dimension "d29" = 2
  dimension "d30" = 9
  dimension "d31" = 1
  constraint midpoint L0 L1.start
  constraint midpoint A0 L1.end
  constraint perpendicular L1 L2
  constraint perpendicular L2 L3
  constraint perpendicular L1 L4
  constraint perpendicular L4 L5
  constraint perpendicular L1 L6
  measures "d27" distance of L1.start L2.end
  measures "d28" distance of L2.end L3.end
  measures "d29" distance of L3.end L4.end
  measures "d30" distance of L4.end L5.end
  measures "d31" distance of L5.end L1.start
extrude "Extrude5" add sketch "Sketch5" along normal blind 3 contours L0 L1 L2 L3 L4 | L0 L1 L4 L5 L6
fillet "Fillet1" radius 1 2 edges at (24.5, 22, -1) (24.5, 22, 1)
mirror "Mirror3" about plane through (0, 0, 0) normal (0, 1, 0) of "Extrude5", "Fillet1"
sketch "Sketch6" plane through (52.4338, 0, 0) normal (1, 0, 0) x (0, 0, -1)
  line L0 (23.5, 13) -> (-23.5, 13)
  line L1 (-23.5, 13) -> (-23.5, 9)
  line L2 (-23.5, 9) -> (23.5, 9)
  line L3 (23.5, 9) -> (23.5, 13)
  line L4 (8, -13) -> (-8, -13)
  line L5 (-8, -13) -> (-8, 13)
  line L6 (-8, 13) -> (8, 13)
  line L7 (8, 13) -> (8, -13)
  line L8 (8, -13) -> (-8, 13) construction
  line L9 (-8, -13) -> (8, 13) construction
  constraint horizontal L4
  constraint perpendicular L4 L5
  constraint parallel L4 L6
  constraint parallel L5 L7
  constraint coincident L8 origin
  constraint coincident L9 origin
extrude "Extrude6" add sketch "Sketch6" along normal blind 3 contours L0 L2 L5 L6 L7 | L2 L4 L5 L7
sketch "Sketch7" plane through (0, 0, 0) normal (-1, 0, 0) x (0, 0, 1)
  circle A0 centre (0, 0) radius 35
  circle A1 centre (0, 0) radius 10
  dimension "d40" = 20
  constraint concentric A0 A1
  measures "d40" diameter of A1
extrude "Extrude7" cut sketch "Sketch7" against normal blind 10 contours A1

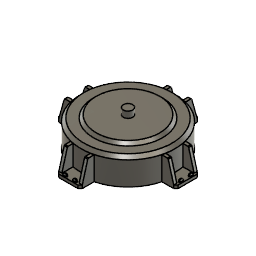
design "BASE"
part number: 2026-02-22-23-03-54-402
Autodesk Fusion 360 part; units mm, degrees
sketch "Sketch1" plane through (0, 0, 0) normal (0, 1, 0) x (1, 0, 0)
  circle A0 centre (0, 0) radius 150
  dimension "d1" = 300
  constraint coincident A0.centre origin
  measures "d1" diameter of A0
extrude "Extrude1" add sketch "Sketch1" along normal blind 75
chamfer "Chamfer1" distance 10 angle 45 1 edges at (-139.8491, 75, 54.2423)
sketch "Sketch2" plane through (0, 0, 0) normal (0, 1, 0) x (1, 0, 0)
sketch "Sketch3" plane through (0, 0, 0) normal (0, 1, 0) x (1, 0, 0)
sketch "Sketch4" plane through (0, 0, 0) normal (0, 1, 0) x (1, 0, 0)
  line L0 (-190, 37.5) -> (-140, 37.5)
  line L1 (-140, 37.5) -> (-140, -37.5)
  line L2 (-140, -37.5) -> (-190, -37.5)
  line L3 (-190, -37.5) -> (-190, 37.5)
  line L4 (0, 0) -> (-150, 0)
  dimension "d5" = 75
  dimension "d6" = 50
  constraint horizontal L0
  constraint vertical L1
  constraint horizontal L2
  constraint vertical L3
  constraint coincident L4.start origin
  constraint perpendicular L1 L4
  constraint symmetric L0 L2 L4
  measures "d5" distance of L0.start L2.end
  measures "d6" distance of L0.start L0.end
extrude "Extrude2" add sketch "Sketch4" against normal blind 10
extrude "Extrude3" add 1 faces at (-43.3333, 0, 0) along direction (0, -1, 0) blind 10
chamfer "Chamfer2" distance 7 angle 45 1 edges at (-190, -5, 37.5)
chamfer "Chamfer3" distance 7 angle 45 1 edges at (-190, -5, -37.5)
sketch "Sketch5" plane through (0, 0, 0) normal (0, 1, 0) x (-1, 0, 0)
  line L0 (183, -37.5) -> (190, -30.5)
  line L1 (190, -30.5) -> (190, 30.5)
  line L2 (190, 30.5) -> (183, 37.5)
  line L3 (183, 37.5) -> (145.2369, 37.5)
  arc A0 (145.2369, -37.5) -> (145.2369, 37.5) centre (0, 0) ccw
  line L4 (145.2369, -37.5) -> (183, -37.5)
sketch "Sketch6" plane through (0, 0, -37.5) normal (0, 0, -1) x (-1, 0, 0)
  line L0 (183, -10) -> (183, 0)
  line L1 (183, 0) -> (145.2369, 0)
  line L2 (145.2369, 0) -> (145.2369, -10)
  line L3 (145.2369, -10) -> (183, -10)
  line L4 (145.2369, 0) -> (145.2369, 64.3683)
  line L5 (145.2369, 64.3683) -> (165.15, 64.3683)
  line L6 (165.15, 64.3683) -> (183, 0)
  dimension "d13" = 17.85
  constraint coincident L1.end L2.start
  constraint perpendicular L1 L4
  constraint perpendicular L4 L5
  constraint coincident L0.end L1.start
  measures "d13" horizontal distance of L5.end L0.end
extrude "Extrude4" add sketch "Sketch6" along normal blind 10 contours L1 L4 L5 L6
extrude "Extrude5" cut 1 faces at (-164.4623, 21.4561, -37.5) along direction (0, 0, 1) blind 10
extrude "Extrude6" add 1 faces at (-164.4623, 21.4561, -37.5) along direction (0, 0, 1) blind 10
extrude "Extrude7" cut 1 faces at (-164.4623, 21.4561, -47.5) along direction (0, 0, 1) blind 10
sketch "Sketch7" plane through (-169.932, 47.1239, 0) normal (-0.963634, 0.267226, 0) x (0, 0, 1)
  line L0 (-37.5, 17.8951) -> (-37.5, -48.9023)
  line L1 (-37.5, -48.9023) -> (-27.5, -48.9023)
  line L2 (-27.5, -48.9023) -> (-27.5, 17.8951)
  line L3 (-27.5, 17.8951) -> (-37.5, 17.8951)
sketch "Sketch8" plane through (-169.932, 47.1239, 0) normal (-0.963634, 0.267226, 0) x (0, 0, 1)
sketch "Sketch9" plane through (-169.932, 47.1239, 0) normal (-0.963634, 0.267226, 0) x (0, 0, 1)
  line L0 (-8.6839, -49.0959) -> (-12.1109, -43.0747)
  line L1 (-12.1109, -43.0747) -> (-19.0389, -43.0319)
  line L2 (-19.0389, -43.0319) -> (-22.54, -49.0104)
  line L3 (-22.54, -49.0104) -> (-19.113, -55.0317)
  line L4 (-19.113, -55.0317) -> (-12.1849, -55.0744)
  line L5 (-12.1849, -55.0744) -> (-8.6839, -49.0959)
  line L6 (-27.5, -48.9) -> (-22.54, -49.0104)
  line L7 (-22.54, -49.0104) -> (-15.6119, -49.0532)
  line L8 (-15.6119, -49.0532) -> (-8.6839, -49.0959)
  point P0 (-15.6119, -49.0532)
  dimension "d25" = 6
  dimension "d26" = 4.96
  constraint coincident P0 L7.end
  measures "d25" distance of P0 L5
  measures "d26" horizontal distance of L2.end L6.start
extrude "Extrude8" add sketch "Sketch9" along normal blind 3.5 contours L0 L1 L2 L7 L8
ref_plane "WorkPlane1" through (-164.1184, 27.1841, 0) normal (0, 0, -1) x (1, 0, 0)
mirror "Mirror1" about plane through (-164.1184, 27.1841, 0) normal (0, 0, -1) of "Extrude8"
mirror "Mirror2" about plane through (-164.1184, 27.1841, 0) normal (0, 0, -1) of "Extrude6"
chamfer "Chamfer4" distance 2 angle 45 1 edges at (-165.15, 64.3683, -32.5)
chamfer "Chamfer5" distance 2 angle 45 1 edges at (-165.15, 64.3683, 32.5)
pattern_circular "C-Pattern1" count 4 over 360 about axis through (0, 1.75, 0) along (0, 1, 0) of "Extrude2", "Chamfer2", "Chamfer3", "Extrude4", "Extrude5", "Extrude6", "Extrude7", "Extrude8", "Mirror1", "Mirror2", "Chamfer4", "Chamfer5"
sketch "Sketch10" plane through (0, 75, 0) normal (0, 1, 0) x (-1, 0, 0)
sketch "Sketch11" plane through (0, 75, 0) normal (0, 1, 0) x (-1, 0, 0)
  circle A0 centre (0, 0) radius 110
  dimension "d40" = 220
  constraint coincident A0.centre origin
  measures "d40" diameter of A0
extrude "Extrude9" add sketch "Sketch11" along normal blind 9 draft -45
sketch "Sketch12" plane through (0, 84, 0) normal (0, 1, 0) x (-1, 0, 0)
  circle A0 centre (0, 0) radius 101
  circle A1 centre (0, 0) radius 15
  dimension "d43" = 30
  constraint concentric A0 A1
  measures "d43" diameter of A1
extrude "Extrude10" add sketch "Sketch12" along normal blind 20 contours A1
named bodies: "BASE"

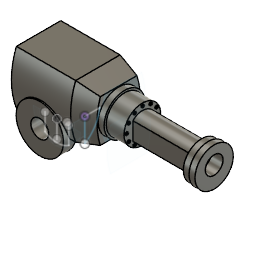
design "JAW 3:1"
part number: 2026-02-28-21-34-13-161
Autodesk Fusion 360 part; units mm, degrees
sketch "Sketch1" plane through (0, 0, 0) normal (1, 0, 0) x (0, 0, -1)
  line L0 (0, 0) -> (0, 45)
  line L1 (0, 0) -> (0, -45)
  line L2 (0, 45) -> (37.5, 45)
  line L3 (0, 45) -> (-37.5, 45)
  line L4 (0, -45) -> (37.5, -45)
  line L5 (0, -45) -> (-37.5, -45)
  arc A0 (-37.5, 45) -> (-37.5, -45) centre (79.119, 0) ccw
  arc A1 (37.5, -45) -> (37.5, 45) centre (-79.119, 0) ccw
  dimension "d2" = 45
  dimension "d3" = 37.5
  dimension "d4" = 37.5
  dimension "d5" = 37.5
  dimension "d6" = 37.5
  dimension "d7" = 125
  dimension "d8" = 125
  constraint coincident L0.start L1.start
  constraint vertical L0
  constraint parallel L0 L1
  constraint perpendicular L0 L2
  constraint perpendicular L0 L3
  constraint perpendicular L1 L4
  constraint perpendicular L1 L5
  measures "d2" distance of L0.start L1.end
  measures "d3" distance of L0.end L2.end
  measures "d4" distance of L0.end L3.end
  measures "d5" distance of L1.end L4.end
  measures "d6" distance of L1.end L5.end
  measures "d7" radius of A1
  measures "d8" radius of A0
extrude "Extrude1" add sketch "Sketch1" along normal blind 100
move_face "MoveFace1" to x (1, 0, 0) y (0, 1, 0) z (0, 0, 1) at (0, 46, 0) 7 faces at (33.3333, 39.2218, -39.5682) (33.3333, 45, -12.5) (66.6667, 45, 25) (66.6667, -45, 12.5) (66.6667, -45, -12.5) (0, -3.0661, -15.1807) (33.3333, 15.306, 44.9403)
extrude "Extrude2" add 1 faces at (100, 42.9339, -15.1807) along direction (1, 0, 0) blind 35 draft -15
sketch "Sketch2" plane through (135, 0, 0) normal (1, 0, 0) x (0, 0, -1)
  line L0 (-30.8786, 10.3782) -> (30.8786, 10.3782)
  arc A0 (30.8786, 10.3782) -> (30.8786, 81.6218) centre (-79.119, 46) ccw
  line L1 (30.8786, 81.6218) -> (-30.8786, 81.6218)
  arc A1 (-30.8786, 81.6218) -> (-30.8786, 10.3782) centre (79.119, 46) ccw
move_body "Move1" bodies 1 to x (1, 0, 0) y (0, 1, 0) z (0, 0, 1) at (0, -51.1307, -9.0041)
sketch "Sketch3" plane through (135, 0, 0) normal (1, 0, 0) x (0, 0, -1)
  line L0 (-21.8745, -40.7524) -> (39.8828, -40.7524)
  arc A0 (39.8828, -40.7524) -> (39.8828, 30.4911) centre (-70.1149, -5.1307) ccw
  line L1 (39.8828, 30.4911) -> (-21.8745, 30.4911)
  arc A1 (-21.8745, 30.4911) -> (-21.8745, -40.7524) centre (88.1232, -5.1307) ccw
move_body "Move2" bodies 1 to x (1, 0, 0) y (0, 1, 0) z (0, 0, 1) at (0, 7.3963, 5.7884)
sketch "Sketch4" plane through (135, 0, 0) normal (1, 0, 0) x (0, 0, -1)
move_body "Move3" bodies 1 to x (1, 0, 0) y (0, 1, 0) z (0, 0, 1) at (0, -2.251, 3.2158)
sketch "Sketch5" plane through (135, 0, 0) normal (1, 0, 0) x (0, 0, -1)
  circle A0 centre (0, 0) radius 34.5
  dimension "d13" = 69
  constraint coincident A0.centre origin
  measures "d13" diameter of A0
extrude "Extrude3" add sketch "Sketch5" along normal blind 10
sketch "Sketch6" plane through (145, 0, 0) normal (1, 0, 0) x (0, 0, -1)
  circle A0 centre (0, 0) radius 34.5
  circle A1 centre (0, 0) radius 31
  dimension "d16" = 62
  constraint concentric A0 A1
  measures "d16" diameter of A1
extrude "Extrude4" add sketch "Sketch6" along normal blind 30 contours A1
sketch "Sketch7" plane through (175, 0, 0) normal (1, 0, 0) x (0, 0, -1)
  circle A0 centre (0, 0) radius 31
  line L0 (0, 0) -> (27, 0)
  circle A1 centre (27, 0) radius 2.5
  circle A2 centre (27, 0) radius 1.5
  dimension "d19" = 27
  dimension "d20" = 5
  dimension "d21" = -1
  constraint coincident A0.centre L0.start
  constraint horizontal L0
  constraint coincident L0.end A1.centre
  measures "d19" distance of A0.centre L0.end
  measures "d20" diameter of A1
extrude "Extrude5" add sketch "Sketch7" along normal blind 1 contours A1
move_body "Move4" bodies 1 to x (1, 0, 0) y (0, 1, 0) z (0, 0, 1) at (0, 45, 0)
pattern_circular "C-Pattern1" count 12 over 360 about axis through (175, 45, 0) along (1, 0, 0) of 2 faces at (176, 45.1242, -29.1574) (175.6667, 45.2489, -29.4876)
sketch "Sketch8" plane through (175, 0, 0) normal (1, 0, 0) x (0, 0, -1)
  circle A0 centre (23.3827, 31.5) radius 2.5
  circle A1 centre (13.5, 21.6173) radius 2.5
  circle A2 centre (0, 18) radius 2.5
  circle A3 centre (-13.5, 21.6173) radius 2.5
  circle A4 centre (-23.3827, 31.5) radius 2.5
  circle A5 centre (-27, 45) radius 2.5
  circle A6 centre (-23.3827, 58.5) radius 2.5
  circle A7 centre (-13.5, 68.3827) radius 2.5
  circle A8 centre (0, 72) radius 2.5
  circle A9 centre (13.5, 68.3827) radius 2.5
  circle A10 centre (23.3827, 58.5) radius 2.5
  circle A11 centre (0, 45) radius 31
  circle A12 centre (27, 45) radius 2.5
  line L0 (0, 45) -> (16, 45)
  line L1 (16, 45) -> (16, 58.1645)
  line L2 (16, 45) -> (16, 28)
  line L3 (0, 45) -> (0, 37)
  line L4 (-16, 45) -> (-16, 58.1645)
  line L5 (-16, 45) -> (-16, 28)
  arc A13 (16, 58.1645) -> (-16, 58.1645) centre (0, 43.0649) ccw
  arc A14 (-16, 28) -> (16, 28) centre (0, 48.4973) ccw
  dimension "d26" = 16
  dimension "d28" = 13.1645
  dimension "d29" = 17
  dimension "d31" = 22
  constraint coincident A11.centre L0.start
  constraint horizontal L0
  constraint perpendicular L0 L1
  constraint perpendicular L0 L2
  constraint perpendicular L0 L3
  constraint symmetric L0.end L3 L4.start
  constraint symmetric L1.end L3 L4.end
  constraint symmetric L2.end L3 L5.end
  constraint tangent A8 A14
  measures "d26" distance of A11.centre L0.end
  measures "d28" distance of L0.end L1.end
  measures "d29" distance of L0.end L2.end
  measures "d31" radius of A13
extrude "Extrude6" add sketch "Sketch8" along normal blind 100 contours L1 L2 L4 L5 A13 A14
sketch "Sketch9" plane through (275, 0, 0) normal (1, 0, 0) x (0, 0, -1)
  line L0 (-16, 58.1645) -> (-16, 28)
  arc A0 (-16, 28) -> (16, 28) centre (0, 48.4973) ccw
  line L1 (16, 28) -> (16, 58.1645)
  arc A1 (16, 58.1645) -> (-16, 58.1645) centre (0, 43.0649) ccw
  circle A2 centre (0, 43.0649) radius 31.0651
  constraint concentric A1 A2
extrude "Extrude7" add sketch "Sketch9" along normal blind 10 contours L0 A0 L1 A1 | A2
sketch "Sketch10" plane through (285, 0, 0) normal (1, 0, 0) x (0, 0, -1)
  circle A0 centre (0, 43.0649) radius 31.0651
  circle A1 centre (0, 43.0649) radius 30.0651
  dimension "d37" = -1
extrude "Extrude8" add sketch "Sketch10" along normal blind 1 contours A1
sketch "Sketch11" plane through (286, 0, 0) normal (1, 0, 0) x (0, 0, -1)
  circle A0 centre (0, 43.0649) radius 30.0651
  circle A1 centre (0, 43.0649) radius 32.384
  constraint concentric A0 A1
extrude "Extrude9" add sketch "Sketch11" along normal blind 10 contours A0 | A1
ref_plane "WorkPlane1" through (0, 90.0146, 37.5) normal (0, 0, 1) x (1, 0, 0)